Kitchen Shelf Cap (Autodesk Fusion 360 design; units mm, degrees)
Autodesk Fusion 360 part; units mm, degrees
sketch "Sketch1" plane through (0, 0, 0) normal (0, 0, 1) x (1, 0, 0)
  line L0 (0, 0) -> (17.6, 0)
  line L1 (17.6, 0) -> (17.6, 38)
  line L2 (17.6, 38) -> (0, 38)
  line L3 (0, 38) -> (0, 0)
  line L4 (-1.5, 0) -> (19.1, 0)
  line L5 (19.1, 0) -> (19.1, 39.5)
  line L6 (19.1, 39.5) -> (-1.5, 39.5)
  line L7 (-1.5, 39.5) -> (-1.5, 0)
  spline S0 degree 2 poles (0, 35.5) (2, 37) (8.8, 38) knots 0 0 0 0.926131 0.926131 0.926131 weights 1 3 1
  spline S1 degree 2 poles (17.6, 35.5) (15.497, 37.1201) (8.8, 38) knots 0 0 0 0.928188 0.928188 0.928188 weights 1 3 1
  dimension "d1" = 38
  dimension "d2" = 17.6
  dimension "d3" = 1.5
  dimension "d4" = 1.5
  dimension "d5" = 1.5
  dimension "d15" = 2.5
  dimension "d16" = 8.8
  dimension "d17" = 8.8
  dimension "d18" = 2.5
  constraint horizontal L0
  constraint vertical L1
  constraint horizontal L2
  constraint vertical L3
  constraint coincident L0.start L3.end
  constraint horizontal L4
  constraint vertical L5
  constraint horizontal L6
  constraint vertical L7
  constraint coincident L2 S0.end
  constraint coincident L3 S0.start
  constraint coincident L1 S1.start
  measures "d1" distance of L0.start L2.end
  measures "d2" distance of L0.start L0.end
  measures "d3" distance of L3 L7
  measures "d4" distance of L1 L5
  measures "d5" distance of L2 L6
  measures "d15" distance of L2.end S0.start
  measures "d16" distance of L2.end S0.end
  measures "d17" distance of L1.end S0.end
  measures "d18" distance of L1.end S1.start
extrude "Extrude1" add sketch "Sketch1" along normal blind 1
extrude "Extrude2" add sketch "Sketch1" along normal blind 7.5 contours L1 L2 L3 L4 L5 L6 L7 | L2 L3 S0 | L1 L2 S1
fillet "Fillet1" radius 4.5 2 edges at (19.1, 39.5, 3.75) (-1.5, 39.5, 3.75)
